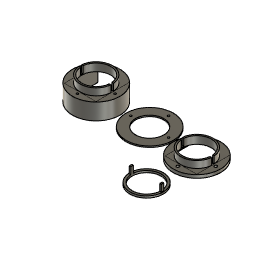
Glass_Stack_holder v8 (Autodesk Fusion 360 design; units mm, degrees)
Autodesk Fusion 360 part; units mm, degrees
sketch "Sketch1" plane through (0, 0, 0) normal (0, 0, 1) x (1, 0, 0)
  line L0 (0, 0) -> (65, 0)
  line L1 (65, 0) -> (65, 65)
  line L2 (65, 65) -> (0, 65)
  line L3 (0, 65) -> (0, 0)
  dimension "d1" = 65
  dimension "d2" = 65
  constraint horizontal L0
  constraint vertical L1
  constraint horizontal L2
  constraint vertical L3
  constraint coincident L0.start L3.end
  measures "d1" distance of L0.start L0.end
  measures "d2" distance of L0.start L2.end
sketch "Sketch2" plane through (0, 0, 2) normal (0, 0, 1) x (-1, 0, 0)
  line L0 (0, -65) -> (0, 0)
  line L1 (0, 0) -> (-65, 0)
  line L2 (-65, 0) -> (-65, -65)
  line L3 (-65, -65) -> (0, -65)
  line L4 (-10, -55) -> (-55, -55)
  line L5 (-55, -55) -> (-55, -10)
  line L6 (-55, -10) -> (-10, -10)
  line L7 (-10, -10) -> (-10, -55)
  dimension "d5" = 45
  dimension "d6" = 45
  constraint horizontal L4
  constraint vertical L5
  constraint horizontal L6
  constraint vertical L7
  measures "d5" distance of L4.start L4.end
  measures "d6" distance of L4.start L6.end
sketch "Sketch3" plane through (0, 0, 2) normal (0, 0, 1) x (-1, 0, 0)
  line L0 (-55, -55) -> (-55, -10)
  line L1 (-55, -10) -> (-10, -10)
  line L2 (-10, -10) -> (-10, -55)
  line L3 (-10, -55) -> (-55, -55)
  line L4 (0, -65) -> (0, 0)
  line L5 (0, 0) -> (-65, 0)
  line L6 (-65, 0) -> (-65, -65)
  line L7 (-65, -65) -> (0, -65)
  line L8 (-7.0093, -58.1542) -> (-58.0093, -58.1542)
  line L9 (-58.0093, -58.1542) -> (-58.0093, -7.1542)
  line L10 (-58.0093, -7.1542) -> (-7.0093, -7.1542)
  line L11 (-7.0093, -7.1542) -> (-7.0093, -58.1542)
  dimension "d9" = 51
  dimension "d10" = 51
  constraint horizontal L8
  constraint vertical L9
  constraint horizontal L10
  constraint vertical L11
  measures "d9" distance of L8.start L8.end
  measures "d10" distance of L8.start L10.end
sketch "Sketch4" plane through (0, 0, 2) normal (0, 0, 1) x (-1, 0, 0)
sketch "Sketch5" plane through (0, 0, 0) normal (0, 0, 1) x (1, 0, 0)
  line L0 (0, 0) -> (70, 0)
  line L1 (70, 0) -> (70, -70)
  line L2 (70, -70) -> (0, -70)
  line L3 (0, -70) -> (0, 0)
  dimension "d23" = 70
  dimension "d24" = 70
  constraint horizontal L0
  constraint vertical L1
  constraint horizontal L2
  constraint vertical L3
  constraint coincident L0.start L3.end
  measures "d23" distance of L0.start L0.end
  measures "d24" distance of L0.start L2.end
sketch "Sketch6" plane through (0, 0, 2) normal (0, 0, 1) x (-1, 0, 0)
  line L0 (0, 70) -> (-70, 70)
  line L1 (-70, 70) -> (-70, 0)
  line L2 (-70, 0) -> (0, 0)
  line L3 (0, 0) -> (0, 70)
  line L4 (-1.5, 1.5) -> (-69, 1.5)
  line L5 (-69, 1.5) -> (-69, 71.5)
  line L6 (-69, 71.5) -> (-1.5, 71.5)
  line L7 (-1.5, 71.5) -> (-1.5, 1.5)
  dimension "d27" = 70
  constraint horizontal L4
  constraint vertical L5
  constraint horizontal L6
  constraint vertical L7
  measures "d27" distance of L4.start L6.end
sketch "Sketch7" plane through (0, 0, 0) normal (0, 0, 1) x (1, 0, 0)
sketch "Sketch8" plane through (0, 0, 2) normal (0, 0, 1) x (-1, 0, 0)
  line L0 (-69, 70) -> (-69, 1.5)
  line L1 (-69, 1.5) -> (-1.5, 1.5)
  line L2 (-1.5, 1.5) -> (-1.5, 70)
  line L3 (-1.5, 70) -> (-69, 70)
  circle A0 centre (-35, 35) radius 49.4975
sketch "Sketch9" plane through (0, 0, 2) normal (0, 0, 1) x (-1, 0, 0)
  line L0 (-70, 70) -> (-69, 70)
  arc A0 (0, 70) -> (-70, 70) centre (-35, 35) ccw
  circle A1 centre (-35, 40) radius 25.5
  line L1 (-60.5371, 15.179) -> (-9.5371, 15.179)
  line L2 (-9.5371, 15.179) -> (-9.5371, 66.179)
  line L3 (-9.5371, 66.179) -> (-60.5371, 66.179)
  line L4 (-60.5371, 66.179) -> (-60.5371, 15.179)
  line L5 (-69, 70) -> (-1.5, 70)
  line L6 (-1.5, 70) -> (0, 70)
  dimension "d34" = 51
  dimension "d35" = 51
  dimension "d36" = 51
  constraint horizontal L1
  constraint vertical L2
  constraint horizontal L3
  constraint vertical L4
  measures "d34" diameter of A1
  measures "d35" distance of L1.start L1.end
  measures "d36" distance of L1.start L3.end
sketch "Sketch10" plane through (0, 0, 1) normal (0, 0, 1) x (-1, 0, 0)
  line L0 (-60.5371, 66.179) -> (-60.5371, 15.179)
  line L1 (-60.5371, 15.179) -> (-9.5371, 15.179)
  line L2 (-9.5371, 15.179) -> (-9.5371, 66.179)
  line L3 (-9.5371, 66.179) -> (-60.5371, 66.179)
  line L4 (-12.8517, 18.2097) -> (-57.8517, 18.2097)
  line L5 (-57.8517, 18.2097) -> (-57.8517, 63.2097)
  line L6 (-57.8517, 63.2097) -> (-12.8517, 63.2097)
  line L7 (-12.8517, 63.2097) -> (-12.8517, 18.2097)
  dimension "d39" = 45
  dimension "d40" = 45
  constraint horizontal L4
  constraint vertical L5
  constraint horizontal L6
  constraint vertical L7
  measures "d39" distance of L4.start L4.end
  measures "d40" distance of L4.start L6.end
sketch "Sketch11" plane through (0, 0, 0) normal (0, 0, 1) x (1, 0, 0)
  line L0 (0, 50) -> (50.5, 50)
  line L1 (50.5, 50) -> (50.5, 100.5)
  line L2 (50.5, 100.5) -> (0, 100.5)
  line L3 (0, 100.5) -> (0, 50)
  dimension "d43" = 50.5
  dimension "d44" = 50.5
  constraint horizontal L0
  constraint vertical L1
  constraint horizontal L2
  constraint vertical L3
  measures "d43" distance of L0.start L0.end
  measures "d44" distance of L0.start L2.end
sketch "Sketch12" plane through (0, 0, 0) normal (0, 0, 1) x (1, 0, 0)
  circle A0 centre (25, 75) radius 37.5
  dimension "d45" = 75
  measures "d45" diameter of A0
extrude "Extrude11" add sketch "Sketch12" along normal blind 2 makes body 1
extrude "Extrude12" add sketch "Sketch11" against normal blind 1 bodies 1
sketch "Sketch13" plane through (0, 0, 2) normal (0, 0, 1) x (-1, 0, 0)
  circle A0 centre (-25, -75) radius 37.5
  line L0 (-25, -75) -> (-50, -75)
  line L1 (-50, -75) -> (-50, -100)
  line L2 (-50, -100) -> (-25, -100)
  line L3 (-25, -100) -> (-25, -75)
  line L4 (-50, -100) -> (0, -100)
  line L5 (0, -100) -> (0, -50)
  line L6 (0, -50) -> (-50, -50)
  line L7 (-50, -50) -> (-50, -100)
  dimension "d50" = 25
  dimension "d51" = 25
  dimension "d52" = 50
  dimension "d53" = 50
  constraint horizontal L0
  constraint vertical L1
  constraint horizontal L2
  constraint vertical L3
  constraint coincident A0.centre L0.start
  constraint horizontal L4
  constraint vertical L5
  constraint horizontal L6
  constraint vertical L7
  measures "d50" distance of A0.centre L0.end
  measures "d51" distance of A0.centre L2.end
  measures "d52" distance of L1.end L4.end
  measures "d53" distance of L1.end L6.end
extrude "Extrude13" cut sketch "Sketch13" against normal blind 1 contours L0 L1 L2 L3 L4 L7 | L0 L3 L4 L5 L6 L7 bodies 1
sketch "Sketch14" plane through (0, 0, 1) normal (0, 0, 1) x (-1, 0, 0)
  line L0 (-50, -50) -> (-50, -100)
  line L1 (-50, -100) -> (0, -100)
  line L2 (0, -100) -> (0, -50)
  line L3 (0, -50) -> (-50, -50)
  circle A0 centre (-25, -75) radius 22.5
  dimension "d56" = 45
  measures "d56" diameter of A0
extrude "Extrude14" cut sketch "Sketch14" against normal blind 10 contours A0 bodies 1
sketch "Sketch15" plane through (0, 0, 2) normal (0, 0, 1) x (-1, 0, 0)
  line L0 (0, -100) -> (-50, -100)
  line L1 (-50, -100) -> (-50, -50)
  line L2 (-50, -50) -> (0, -50)
  line L3 (0, -50) -> (0, -100)
  circle A0 centre (-25, -75) radius 37.5
  line L4 (0, -50) -> (0, -47.0492)
  line L5 (-50, -50) -> (-50, -47.0492)
  constraint coincident L2.end L3.start
  constraint coincident A0 L4.end
  constraint perpendicular L2 L4
  constraint coincident L1.end L2.start
  constraint coincident A0 L5.end
  constraint perpendicular L2 L5
extrude "Extrude15" cut sketch "Sketch15" against normal blind 1 contours L2 A0 L4 L5 bodies 1
extrude "Extrude16" cut 1 faces at (33.3333, 100, 1.3333) along direction (0, 1, 0) blind 0.5 on bodies 1 bodies 1
extrude "Extrude17" cut 1 faces at (50, 82.6831, 1.6667) along direction (1, 0, 0) blind 0.2 on bodies 1 bodies 1
extrude "Extrude18" cut 1 faces at (0, 82.6831, 1.6667) along direction (-1, 0, 0) blind 0.2 on bodies 1 bodies 1
extrude "Extrude19" add 1 faces at (24.3897, 104.4851, 2) along direction (0, 0, 1) blind 23 on bodies 1 bodies 1
extrude "Extrude21" add 1 faces at (24.6062, 99.479, -1) along direction (0, 0, -1) blind 1 on bodies 1 bodies 1
extrude "Extrude22" cut 1 faces at (24.6062, 99.479, -2) along direction (0, 0, 1) blind 2 on bodies 1 bodies 1
sketch "Sketch19" plane through (0, 0, 25) normal (0, 0, 1) x (-1, 0, 0)
  line L0 (0.2, -47.2293) -> (0.2, -100.5)
  line L1 (0.2, -100.5) -> (-50.2, -100.5)
  line L2 (-50.2, -100.5) -> (-50.2, -47.2293)
  arc A0 (-50.2, -47.2293) -> (0.2, -47.2293) centre (-25, -75) ccw
  circle A1 centre (5, -75) radius 1.55
  circle A2 centre (-25, -105) radius 1.55
  circle A3 centre (-55, -75) radius 1.55
  dimension "d83" = 3.1
  dimension "d84" = 3.1
  dimension "d85" = 3.1
  measures "d83" diameter of A1
  measures "d84" diameter of A2
  measures "d85" diameter of A3
extrude "Extrude24" cut sketch "Sketch19" against normal blind 35 contours A1 | A2 | A3 bodies 1
extrude "Extrude25" add 1 faces at (-4.0995, 89.8008, 25) along direction (0, 0, 1) blind 1 on bodies 1 bodies 1
sketch "Sketch20" plane through (0, 0, 0) normal (0, 0, 1) x (1, 0, 0)
  circle A0 centre (125, 80) radius 37.5
  dimension "d90" = 75
  measures "d90" diameter of A0
extrude "Extrude26" add sketch "Sketch20" along normal blind 2 separate body makes body 2
sketch "Sketch21" plane through (0, 0, 2) normal (0, 0, 1) x (-1, 0, 0)
  circle A0 centre (-125, -80) radius 37.5
  circle A1 centre (-125, -80) radius 22.5
  dimension "d93" = 45
  constraint concentric A0 A1
  measures "d93" diameter of A1
extrude "Extrude27" cut sketch "Sketch21" against normal blind 5 contours A1 bodies 2
sketch "Sketch22" plane through (0, 0, 2) normal (0, 0, 1) x (-1, 0, 0)
  circle A0 centre (-125, -80) radius 22.5
  circle A1 centre (-125, -80) radius 37.5
  circle A2 centre (-125, -110) radius 1.55
  circle A3 centre (-95, -80) radius 1.55
  circle A4 centre (-155, -80) radius 1.55
  dimension "d96" = 3.1
  dimension "d97" = 3.1
  dimension "d98" = 3.1
  measures "d96" diameter of A2
  measures "d97" diameter of A3
  measures "d98" diameter of A4
extrude "Extrude28" cut sketch "Sketch22" against normal blind 5 contours A2 | A3 | A4 bodies 2
copy_body "CopyPasteBodies1" bodies 1 makes body 3
move_body "Move1" bodies 3 to x (1, 0, 0) y (0, 1, 0) z (0, 0, 1) at (185, 0, 0)
extrude "Extrude29" cut 1 faces at (180.9005, 89.8008, 26) along direction (0, 0, -1) blind 21 on bodies 3 bodies 3
move_body "Move2" bodies 1 to x (1, 0, 0) y (0, 1, 0) z (0, 0, 1) at (20, 0, 0)
move_body "Move3" bodies 3 to x (1, 0, 0) y (0, 1, 0) z (0, 0, 1) at (-5, 0, 0)
sketch "Sketch23" plane through (0, 0, 26) normal (0, 0, 1) x (-1, 0, 0)
  circle A0 centre (-45, -105) radius 1.55
  circle A1 centre (-15, -75) radius 1.55
  circle A2 centre (-75, -75) radius 1.55
  line L0 (-19.8, -47.2293) -> (-19.8, -100.5)
  line L1 (-19.8, -100.5) -> (-70.2, -100.5)
  line L2 (-70.2, -100.5) -> (-70.2, -47.2293)
  arc A3 (-70.2, -47.2293) -> (-19.8, -47.2293) centre (-45, -75) ccw
  circle A4 centre (-15, -75) radius 2.25
  circle A5 centre (-45, -105) radius 2.25
  circle A6 centre (-75, -75) radius 2.25
  dimension "d103" = 4.5
  dimension "d104" = 4.5
  dimension "d105" = 4.5
  constraint concentric A1 A4
  constraint concentric A0 A5
  constraint concentric A2 A6
  measures "d103" diameter of A4
  measures "d104" diameter of A5
  measures "d105" diameter of A6
extrude "Extrude30" cut sketch "Sketch23" against normal blind 6 contours A4 | A5 | A6 bodies 1
sketch "Sketch24" plane through (0, 0, 5) normal (0, 0, 1) x (-1, 0, 0)
  circle A0 centre (-205, -105) radius 1.55
  circle A1 centre (-175, -75) radius 1.55
  circle A2 centre (-235, -75) radius 1.55
  line L0 (-179.8, -47.2293) -> (-179.8, -100.5)
  line L1 (-179.8, -100.5) -> (-230.2, -100.5)
  line L2 (-230.2, -100.5) -> (-230.2, -47.2293)
  arc A3 (-230.2, -47.2293) -> (-179.8, -47.2293) centre (-205, -75) ccw
  circle A4 centre (-175, -75) radius 2.25
  circle A5 centre (-205, -105) radius 2.25
  circle A6 centre (-235, -75) radius 2.25
  dimension "d108" = 4.5
  dimension "d109" = 4.5
  dimension "d110" = 4.5
  constraint concentric A1 A4
  constraint concentric A0 A5
  constraint concentric A2 A6
  measures "d108" diameter of A4
  measures "d109" diameter of A5
  measures "d110" diameter of A6
extrude "Extrude31" cut sketch "Sketch24" against normal blind 6 contours A4 | A5 | A6 bodies 3
move_body "Move4" bodies 1 to x (1, 0, 0) y (0, -1, 0) z (0, 0, -1) at (0, 150, 0)
sketch "Sketch25" plane through (0, 0, 0) normal (0, 0, 1) x (-1, 0, 0)
  circle A0 centre (-45, -45) radius 1.55
  circle A1 centre (-15, -75) radius 1.55
  circle A2 centre (-75, -75) radius 1.55
  circle A3 centre (-45, -75) radius 22.5
  circle A4 centre (-45, -75) radius 37.5
  circle A5 centre (-45, -75) radius 10
  circle A6 centre (-45, -75) radius 27.5
  dimension "d113" = 20
  dimension "d114" = 55
  constraint concentric A3 A5
  constraint concentric A5 A6
  measures "d113" diameter of A5
  measures "d114" diameter of A6
extrude "Extrude32" add sketch "Sketch25" along normal blind 5 contours A3 | A6 bodies 1
sketch "Sketch26" plane through (0, 0, 5) normal (0, 0, 1) x (-1, 0, 0)
  circle A0 centre (-45, -75) radius 10
  circle A1 centre (-45, -75) radius 27.5
  circle A2 centre (-45, -75) radius 8
  dimension "d117" = 16
  constraint concentric A0 A2
  measures "d117" diameter of A2
extrude "Extrude33" add sketch "Sketch26" along normal blind 10 separate body contours A0 makes body 4
extrude "Extrude34" add 1 faces at (35.7039, 75.4968, 5) along direction (0, 0, -1) blind 5 on bodies 4 bodies 1 4
extrude "Extrude35" add 1 faces at (27.4469, 73.4847, 0) along direction (0, 0, -1) blind 1 on bodies 1 bodies 1
move_body "Move5" bodies 3 to x (1, 0, 0) y (0, -1, 0) z (0, 0, -1) at (0, 150, 0)
sketch "Sketch27" plane through (0, 0, 0) normal (0, 0, 1) x (-1, 0, 0)
  circle A0 centre (-175, -75) radius 2.25
  circle A1 centre (-205, -45) radius 2.25
  circle A2 centre (-235, -75) radius 2.25
  circle A3 centre (-205, -75) radius 22.5
  circle A4 centre (-205, -75) radius 37.5
  circle A5 centre (-205, -75) radius 27.5
  dimension "d124" = 55
  constraint concentric A3 A5
  measures "d124" diameter of A5
extrude "Extrude36" add sketch "Sketch27" along normal blind 5 contours A3 | A5 bodies 3
sketch "Sketch28" plane through (0, 0, 5) normal (0, 0, 1) x (-1, 0, 0)
  circle A0 centre (-205, -75) radius 27.5
  circle A1 centre (-205, -75) radius 10
  circle A2 centre (-205, -75) radius 8
  dimension "d127" = 20
  dimension "d128" = 16
  constraint concentric A0 A1
  constraint concentric A1 A2
  measures "d127" diameter of A1
  measures "d128" diameter of A2
extrude "Extrude37" add sketch "Sketch28" along normal blind 10 contours A1 bodies 3
extrude "Extrude38" cut 1 faces at (209.5917, 72.7888, 5) along direction (0, 0, -1) blind 20 on bodies 3 bodies 3
extrude "Extrude39" add 1 faces at (187.4469, 73.4847, 0) along direction (0, 0, -1) blind 1 on bodies 3 bodies 3
move_body "Move6" bodies 1 to x (1, 0, 0) y (0, 1, 0) z (0, 0, 1) at (0, 0, 25)
move_body "Move7" bodies 3 to x (1, 0, 0) y (0, 1, 0) z (0, 0, 1) at (0, 0, 5)
move_face "OffsetFaces1" offset -2 1 faces at (232.3633, 77.7381, 6.6667) on bodies 3
extrude "Extrude40" cut 1 faces at (195.7337, 75.8943, 20) along direction (0, 0, -1) blind 10 on bodies 3 bodies 3
extrude "Extrude41" add 1 faces at (185.4283, 76.2669, 10) along direction (0, 0, 1) blind 6 on bodies 3 bodies 3
move_face "OffsetFaces2" offset -15 1 faces at (197.0099, 75.3988, 12) on bodies 3
sketch "Sketch29" plane through (0, 0, 16) normal (0, 0, 1) x (-1, 0, 0)
  circle A0 centre (-205, -75) radius 23
  circle A1 centre (-205, -75) radius 25.5
  line L0 (-235, -75) -> (-175, -75)
  line L1 (-235, -75) -> (-175, -75)
  line L2 (-175, -75) -> (-175, -73)
  line L3 (-175, -73) -> (-235, -73)
  line L4 (-235, -73) -> (-235, -75)
  line L5 (-235, -75) -> (-175, -75)
  line L6 (-175, -75) -> (-175, -77)
  line L7 (-175, -77) -> (-235, -77)
  line L8 (-235, -77) -> (-235, -75)
  constraint horizontal L0
  constraint horizontal L1
  constraint vertical L2
  constraint horizontal L3
  constraint vertical L4
  constraint horizontal L5
  constraint vertical L6
  constraint horizontal L7
  constraint vertical L8
extrude "Extrude42" cut sketch "Sketch29" against normal blind 11 contours A0 A1 L0 L1 L5 L7 | A0 A1 L0 L1 L3 L5 | A0 A1 L0 L1 L3 L5 | A0 A1 L0 L1 L5 L7 bodies 3
sketch "Sketch30" plane through (0, 0, 0) normal (0, 0, 1) x (1, 0, 0)
  circle A0 centre (200, -25) radius 25.5
  dimension "d143" = 51
  measures "d143" diameter of A0
extrude "Extrude43" add sketch "Sketch30" along normal blind 3 separate body makes body 5
sketch "Sketch31" plane through (0, 0, 3) normal (0, 0, 1) x (-1, 0, 0)
  circle A0 centre (-200, 25) radius 25.5
  circle A1 centre (-200, 25) radius 23
  dimension "d146" = 46
  constraint concentric A0 A1
  measures "d146" diameter of A1
extrude "Extrude44" cut sketch "Sketch31" against normal blind 5 contours A1 bodies 5
move_body "Move8" bodies 5 to x (1, 0, 0) y (0, 1, 0) z (0, 0, 1) at (0, 25, 0)
sketch "Sketch32" plane through (0, 0, 3) normal (0, 0, 1) x (-1, 0, 0)
  circle A0 centre (-200, 0) radius 23
  circle A1 centre (-200, 0) radius 25.5
  line L0 (-227, 0) -> (-173, 0)
  line L1 (-227, 0) -> (-173, 0)
  line L2 (-173, 0) -> (-173, 2)
  line L3 (-173, 2) -> (-227, 2)
  line L4 (-227, 2) -> (-227, 0)
  line L5 (-227, 0) -> (-173, 0)
  line L6 (-173, 0) -> (-173, -2)
  line L7 (-173, -2) -> (-227, -2)
  line L8 (-227, -2) -> (-227, 0)
  constraint horizontal L0
  constraint horizontal L1
  constraint vertical L2
  constraint horizontal L3
  constraint vertical L4
  constraint horizontal L5
  constraint vertical L6
  constraint horizontal L7
  constraint vertical L8
extrude "Extrude45" add sketch "Sketch32" along normal blind 11 contours A0 A1 L0 L1 L5 L7 | A0 A1 L0 L1 L3 L5 | A0 A1 L0 L1 L3 L5 | A0 A1 L0 L1 L5 L7 bodies 5
sketch "Sketch33" plane through (0, 0, 0) normal (0, 0, 1) x (1, 0, 0)
sketch "Sketch34" plane through (0, 0, 3) normal (0, 0, 1) x (-1, 0, 0)
  line L0 (-177.0871, 2) -> (-174.5786, 2)
  arc A0 (-174.5786, 2) -> (-225.4214, 2) centre (-200, 0) ccw
  line L1 (-225.4214, 2) -> (-222.9129, 2)
  arc A1 (-177.0871, 2) -> (-222.9129, 2) centre (-200, 0) ccw
  circle A2 centre (-200, 0) radius 26.5
  dimension "d151" = 53
  constraint concentric A0 A2
  measures "d151" diameter of A2
extrude "Extrude46" add sketch "Sketch34" against normal blind 3 bodies 5
sketch "Sketch35" plane through (0, 0, 3) normal (0, 0, 1) x (-1, 0, 0)
  line L0 (-177.0871, 2) -> (-174.5786, 2)
  arc A0 (-174.5786, -2) -> (-174.5786, 2) centre (-200, 0) ccw
  line L1 (-174.5786, -2) -> (-177.0871, -2)
  arc A1 (-177.0871, -2) -> (-177.0871, 2) centre (-200, 0) ccw
  circle A2 centre (-200, 0) radius 26.5
  arc A3 (-222.9129, 2) -> (-222.9129, -2) centre (-200, 0) ccw
  line L2 (-222.9129, -2) -> (-225.4214, -2)
  arc A4 (-225.4214, 2) -> (-225.4214, -2) centre (-200, 0) ccw
  line L3 (-225.4214, 2) -> (-222.9129, 2)
  circle A5 centre (-200, 0) radius 23
  dimension "d154" = 46
  constraint concentric A0 A5
  measures "d154" diameter of A5
extrude "Extrude47" cut sketch "Sketch35" against normal blind 10 contours A1 A3 A5 bodies 5
extrude "Extrude48" cut 1 faces at (35.7039, 75.4968, 40) along direction (0, 0, -1) blind 10 on bodies 1 bodies 1
move_face "OffsetFaces3" offset -2 1 faces at (72.3633, 77.7381, 26.6667) on bodies 1
move_face "OffsetFaces4" offset -15 1 faces at (37.0398, 75.7965, 28) on bodies 1
extrude "Extrude49" add 1 faces at (20.4283, 76.2669, 30) along direction (0, 0, 1) blind 6 on bodies 1 bodies 1
sketch "Sketch36" plane through (0, 0, 36) normal (0, 0, 1) x (-1, 0, 0)
  circle A0 centre (-45, -75) radius 23
  circle A1 centre (-45, -75) radius 25.5
  line L0 (-75, -75) -> (-15, -75)
  line L1 (-75, -75) -> (-15, -75)
  line L2 (-15, -75) -> (-15, -73)
  line L3 (-15, -73) -> (-75, -73)
  line L4 (-75, -73) -> (-75, -75)
  line L5 (-75, -75) -> (-15, -75)
  line L6 (-15, -75) -> (-15, -77)
  line L7 (-15, -77) -> (-75, -77)
  line L8 (-75, -77) -> (-75, -75)
  constraint horizontal L0
  constraint horizontal L1
  constraint vertical L2
  constraint horizontal L3
  constraint vertical L4
  constraint horizontal L5
  constraint vertical L6
  constraint horizontal L7
  constraint vertical L8
extrude "Extrude50" cut sketch "Sketch36" against normal blind 11 contours A0 A1 L0 L1 L5 L7 | A0 A1 L0 L1 L3 L5 | A0 A1 L0 L1 L3 L5 | A0 A1 L0 L1 L5 L7 bodies 1
